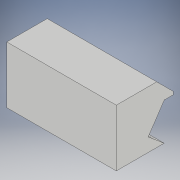
# Autodesk Inventor part: plowV3
Saved by Autodesk Inventor 2019 (Build 230136000, 136)
## iProperties
Created: 2019-04-05
Part Number: plowV3
Material: Generic
Document SubType Name: Modeling
Designer: Tesler
Density: 1 g/cm^3
Appearance: Default
Author: Tesler
Autodesk Inventor part; units mm, degrees
ref_plane "YZ Plane" through (0, 0, 0) normal (1, 0, 0) x (0, 1, 0)
ref_plane "XZ Plane" through (0, 0, 0) normal (0, 1, 0) x (-1, 0, 0)
sketch "Sketch1" plane through (0, 0, 0) normal (1, 0, 0) x (0, 1, 0)
  line L0 (0, 0) -> (95, 0)
  line L1 (95, 0) -> (95, -67.5)
  line L2 (0, 0) -> (0, -80)
  line L3 (0, -80) -> (62.9325, -5)
  line L4 (0, -80) -> (117.6394, -80) construction
  line L5 (67.5, -95) -> (95, -67.5)
  line L6 (90, -5) -> (90, -67.5)
  line L7 (62.5, -95) -> (67.5, -95)
  line L8 (62.5, -95) -> (90, -67.5)
  line L9 (57.9325, -5) -> (5, -68.9585)
  line L10 (5, -5) -> (5, -68.9585)
  line L11 (90, -5) -> (62.9325, -5)
  line L12 (57.9325, -5) -> (5, -5)
  point P0 (0, -75)
  dimension "d0" = 95
  dimension "d2" = 80
  dimension "d5" = 50
  dimension "d22" = 5
  dimension "d23" = 5
  dimension "d24" = 27.5
  dimension "d27" = 5
  dimension "d28" = 5
  dimension "d29" = 5
  dimension "d30" = 50.389
  dimension "d31" = 95
  dimension "d32" = 67.5
  dimension "d34" = 68.9585
  dimension "d35" = 5
  dimension "d36" = 27.5
  constraints: 26 end point, 4 vertical, 3 horizontal, 2 perpendicular, 1 point on line
  measures "d0" distance of L0.start L0.end
  measures "d2" distance of L0.start L2.end
  measures "d5" angle of L4 L3
  measures "d22" distance of L5.start L7.start
  measures "d23" distance between parallel lines of L1 L6
  measures "d24" horizontal distance of L5.start L1.end
  measures "d27" distance of L3.end L9.start
  measures "d28" distance of L2.end point (0, -75)
  measures "d29" distance between parallel lines of L2 L10
  measures "d30" angle of L9 L12
  measures "d31" distance from line of L0 L7.start
  measures "d32" distance from line of L0 L6.end
  measures "d34" distance from line of L9.end L0
  measures "d35" distance between parallel lines of L0 L12
  measures "d36" horizontal distance of L7.start L6.end
extrude "Extrusion1" add sketch "Sketch1" along normal blind 177.8
sketch "Sketch3" plane through (177.8, 0, 0) normal (1, 0, 0) x (0, 0, -1)
  line L0 (0, 95) -> (0, 0) projected
  line L1 (67.5, 95) -> (0, 95) projected
  line L2 (95, 67.5) -> (67.5, 95) projected
  line L3 (0, 0) -> (80, 0) projected
  line L4 (0, 95) -> (67.5, 95)
  line L5 (80, 0) -> (0, 0)
  line L6 (0, 0) -> (0, 95)
  line L7 (80, 0) -> (5, 62.9325) projected
  line L8 (80, 0) -> (53.1884, 22.4976)
  line L9 (53.1884, 22.4976) -> (80, 62.5)
  line L10 (95, 62.5) -> (67.5, 90) projected
  line L11 (95, 62.5) -> (80, 62.5)
  line L12 (67.5, 95) -> (95, 67.5) projected
  line L13 (67.5, 95) -> (95, 67.5)
  line L14 (95, 67.5) -> (95, 62.5)
  line L15 (95, 62.5) -> (95, 67.5)
  dimension "d37" = 35
  dimension "d39" = 15
  dimension "d40" = 40.0024
  constraints: 18 end point, 2 collinear, 2 point on line, 1 horizontal, 1 parallel
  measures "d37" distance of L3.end L8.end
  measures "d39" distance of L10.start L9.end
  measures "d40" vertical distance of L8.end L9.end
extrude "Extrusion2" add sketch "Sketch3" along normal blind 5
ref_plane "Work Plane1" through (91.4, 0, 0) normal (1, 0, 0) x (0, 0, -1)
mirror "Mirror1" about plane through (91.4, 0, 0) normal (1, 0, 0) of "Extrusion2"
body "Solid1"
